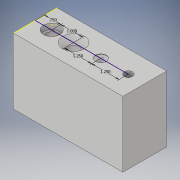
# Autodesk Inventor part: 7.2 part 4
Saved by Autodesk Inventor 2017 (Build 210142000, 142)
## iProperties
Created: 2017-03-16
Part Number: 7.2 part 4
Material: Generic
Document SubType Name: Modeling
Designer: 196918
Density: 1 g/cm^3
Appearance: Default
Author: 196918
Autodesk Inventor part; units mm, degrees
ref_plane "YZ Plane" through (0, 0, 0) normal (1, 0, 0) x (0, 1, 0)
ref_plane "XZ Plane" through (0, 0, 0) normal (0, 1, 0) x (-1, 0, 0)
ref_plane "XY Plane" through (0, 0, 0) normal (0, 0, 1) x (1, 0, 0)
sketch "Sketch1" plane through (0, 0, 0) normal (0, 1, 0) x (-1, 0, 0)
  line L0 (14.2949, 30.3382) -> (-112.7051, 30.3382)
  line L1 (-112.7051, 30.3382) -> (-112.7051, -20.4618)
  line L2 (-112.7051, -20.4618) -> (14.2949, -20.4618)
  line L3 (14.2949, -20.4618) -> (14.2949, 30.3382)
  point P0 (0, 0)
  dimension "d0" = 127
  dimension "d1" = 50.8
  constraints: 8 end point, 2 parallel, 1 horizontal, 1 perpendicular
  measures "d0" distance of L2.end L1.end
  measures "d1" distance of L1.end L0.end
extrude "Extrusion1" add sketch "Sketch1" along normal blind 76.2
sketch "Sketch2" plane through (0, 76.2, 0) normal (0, 1, 0) x (1, 0, 0)
  line L0 (-14.2949, 20.4618) -> (-14.2949, -30.3382) projected
  line L1 (-14.2949, -4.9382) -> (4.7551, -4.9382)
  line L2 (4.7551, -4.9382) -> (30.1551, -4.9382)
  line L3 (30.1551, -4.9382) -> (61.9051, -4.9382)
  line L4 (61.9051, -4.9382) -> (93.6551, -4.9382)
  point P0 (0, 0)
  dimension "d4" = 19.05
  dimension "d5" = 25.4
  dimension "d6" = 31.75
  dimension "d7" = 31.75
  constraints: 8 end point, 4 coincident, 2 horizontal, 2 point on line, 1 midpoint
  measures "d4" distance of L1.start L1.end
  measures "d5" distance of L1.end L2.end
  measures "d6" distance of L2.end L3.end
  measures "d7" distance of L3.end L4.end
hole "Hole1" at (93.6551, 76.2, 4.9382) direction (0, -1, 0) diameter 6.35 depth 25.4 tip angle 118
hole "Hole2" at (93.6551, 76.2, 4.9382) direction (0, -1, 0) diameter 9.525 depth 6.35 tip angle 118
hole "Hole3" at (61.9051, 76.2, 4.9382) direction (0, -1, 0) diameter 12.7 depth 0.508 tip angle 118
hole "Hole4" at (30.1551, 76.2, 4.9382) direction (0, -1, 0) diameter 12.7 depth 76.2 tip angle 118 countersink diameter 25.4 countersink angle 82
hole "Hole5" at (4.7551, 76.2, 4.9382) direction (0, -1, 0) diameter 12.7 depth 76.2 tip angle 118 counterbore diameter 19.05 counterbore depth 6.35
body "Solid1"
